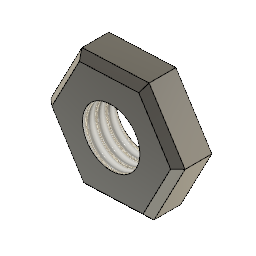
_nut.b28b7be6-7d55-42bf-8755-f202b78b590d (Autodesk Fusion 360 design; units mm, degrees)
Autodesk Fusion 360 part; units mm, degrees
sketch "Sketch1" plane through (0, 0, 0) normal (0, 1, 0) x (1, 0, 0)
  circle A0 centre (0, 0) radius 5
  line L0 (4.6379, -8.8595) -> (9.9915, -0.4132)
  line L1 (9.9915, -0.4132) -> (5.3536, 8.4463)
  line L2 (5.3536, 8.4463) -> (-4.6379, 8.8595)
  line L3 (-4.6379, 8.8595) -> (-9.9915, 0.4132)
  line L4 (-9.9915, 0.4132) -> (-5.3536, -8.4463)
  line L5 (-5.3536, -8.4463) -> (4.6379, -8.8595)
  dimension "d1" = 10
  constraint coincident A0.centre origin
  measures "d1" diameter of A0
extrude "Extrude1" add sketch "Sketch1" along normal blind 5
chamfer "Chamfer1" distance 1 angle 45 6 edges at (-7.3147, 0, -4.6363) (-7.6725, 0, 4.0165) (-0.3578, 0, 8.6529) (7.3147, 0, 4.6363) (7.6725, 0, -4.0165) (0.3578, 0, -8.6529)
thread "Thread1" "ISO Metric profile 10.0 M10x1.5 6H" major diameter 10.198 minor diameter 8.526 pitch 1.5 angle 60 resizes the face on face at (4.9938, 3.3333, 0.2492)
